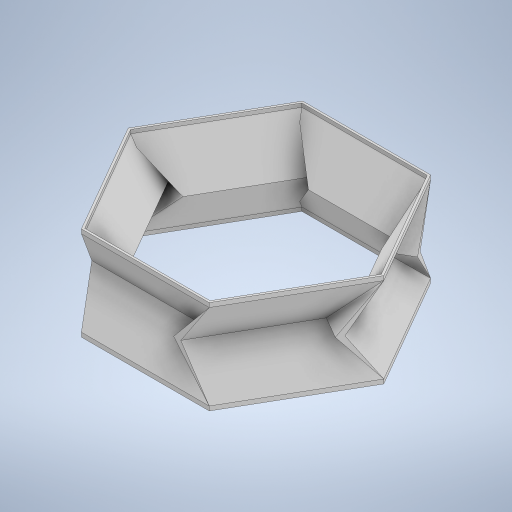
# Autodesk Inventor part: OV-PAM_n_6_standard_1F
Saved by Autodesk Inventor 2024 (Build 280153000, 153)
## iProperties
Created: 2023-08-31
Part Number: OV-PAM_n_6_standard_1F
Material: 일반
Document SubType Name: Modeling
Designer: jsw
Density: 1 g/cm^3
Appearance: 기본값
Author: jsw
Autodesk Inventor part; units mm, degrees
ref_plane "YZ Plane" through (0, 0, 0) normal (1, 0, 0) x (0, 1, 0)
ref_plane "XZ Plane" through (0, 0, 0) normal (0, 1, 0) x (-1, 0, 0)
ref_plane "XY Plane" through (0, 0, 0) normal (0, 0, 1) x (1, 0, 0)
sketch "스케치1" plane through (0, 0, 0) normal (0, 1, 0) x (-1, 0, 0)
  line L0 (17.6385, 30.5508) -> (35.277, 0)
  line L1 (35.277, 0) -> (17.6385, -30.5508)
  line L2 (17.6385, -30.5508) -> (-17.6385, -30.5508)
  line L3 (-17.6385, -30.5508) -> (-35.277, 0)
  line L4 (-35.277, 0) -> (-17.6385, 30.5508)
  line L5 (-17.6385, 30.5508) -> (17.6385, 30.5508)
  line L6 (35.9698, 0) -> (17.9849, -31.1508)
  line L7 (17.9849, -31.1508) -> (-17.9849, -31.1508)
  line L8 (-17.9849, -31.1508) -> (-35.9698, 0)
  line L9 (-35.9698, 0) -> (-17.9849, 31.1508)
  line L10 (-17.9849, 31.1508) -> (17.9849, 31.1508)
  line L11 (17.9849, 31.1508) -> (35.9698, 0)
  point P0 (0, 0)
  point P1 (0, 0)
  point P2 (0, 0)
  dimension "d0" = 70.554
  dimension "d1" = 0.6
  constraints: 24 end point, 2 coincident, 2 horizontal, 26 other
  measures "d0" distance of L3.end L0.end
  measures "d1" distance between parallel lines of L1 L6
extrude "돌출1" add sketch "스케치1" along normal blind 12 contours L0 L1 L2 L3 L4 L5 | L6 L7 L8 L9 L10 L11
ref_plane "작업 평면1" through (17.9849, 0, 31.1508) normal (-0.75, -0.5, -0.4330127) x (0.5, 0, -0.8660254)
sketch "스케치2" plane through (35.9698, 0, 0) normal (0.8660254, 0, 0.5) x (0.5, 0, -0.8660254)
  line L0 (-35.9698, 0) -> (0, 0) projected
  line L1 (0, 0) -> (0, 12) projected
  line L2 (-35.9698, 12) -> (0, 12) projected
  line L3 (-35.9698, 0) -> (-35.9698, 12) projected
  line L4 (-35.9698, 0) -> (-46.039, 12)
  line L5 (-53.9547, 12) -> (-35.9698, 12) projected
  line L6 (0, 0) -> (-10, 12)
  point P0 (-17.9849, 0)
  dimension "d5" = 130
  dimension "d6" = 10
  constraints: 4 end point, 2 point on line
  measures "d5" angle of L4 L0
  measures "d6" distance of L1.end L6.end
extrude "돌출2" cut sketch "스케치2" against normal up to surface contours L3 L2 L6 L0 | L4 L5 L3 surface through (17.9849, 0, 31.1508) normal (-0.75, -0.5, -0.4330127)
pattern_circular "원형 패턴1" count 6 over 360 about axis through (0, -10, 0) along (0, 1, 0) of "돌출2"
ref_plane "작업 평면2" through (0, 12, 0) normal (0, 1, 0) x (1, 0, 0)
sketch "스케치3" plane through (0, 0, 0) normal (0, -1, 0) x (1, 0, 0)
  line L0 (-17.9849, 31.1508) -> (17.9849, 31.1508) projected
  line L1 (-35.9698, 0) -> (-17.9849, 31.1508) projected
  line L2 (-17.9849, -31.1508) -> (-35.9698, 0) projected
  line L3 (17.9849, -31.1508) -> (-17.9849, -31.1508) projected
  line L4 (35.9698, 0) -> (17.9849, -31.1508) projected
  line L5 (17.9849, 31.1508) -> (35.9698, 0) projected
  point P0 (0, 0)
extrude "돌출3" add sketch "스케치3" along normal blind 1.2
mirror "미러1" about plane through (0, 12, 0) normal (0, 1, 0) of "돌출2", "원형 패턴1", "돌출1", "돌출3"
shell "쉘1" thickness 0.6 removed faces 2 at (-11.9899, 25.2, 0) at (-11.9899, -1.2, 0)
